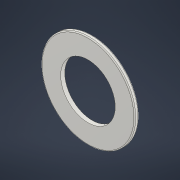
# Autodesk Inventor part: rondelle
Saved by Autodesk Inventor 2022.1 (Build 261234020, 234B)
## iProperties
Created: 2021-12-02
Part Number: rondelle
Material: Generic
Document SubType Name: Modeling
Designer: PaulT
Density: 1 g/cm^3
Appearance: Steel
Author: PaulT
Autodesk Inventor part; units mm, degrees
ref_plane "YZ Plane" through (0, 0, 0) normal (1, 0, 0) x (0, 1, 0)
ref_plane "XZ Plane" through (0, 0, 0) normal (0, 1, 0) x (-1, 0, 0)
ref_plane "XY Plane" through (0, 0, 0) normal (0, 0, 1) x (1, 0, 0)
sketch "Sketch1" plane through (0, 0, 0) normal (0, 0, 1) x (1, 0, 0)
  circle A0 centre (0, 0) radius 5.15
  circle A1 centre (0, 0) radius 3
  dimension "d0" = 6
  dimension "d1" = 10.3
  constraints: 2 centre point, 2 coincident
  measures "d0" diameter of A1
  measures "d1" diameter of A0
extrude "Extrusion1" add sketch "Sketch1" against normal blind 0.45
fillet "Fillet1" radius 0.1 2 edges at (-5.15, 0, 0) (-5.15, 0, -0.45)
body "Solid1"
